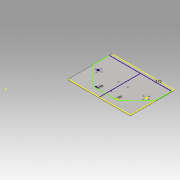
# Autodesk Inventor part: track side panel V1
Saved by Autodesk Inventor 2016 (Build 200138000, 138)
## iProperties
Created: 2015-10-10
Part Number: track side panel V1
Material: Generic
Document SubType Name: Modeling
Designer: Delta
Density: 1 g/cm^3
Appearance: Default
Author: Delta
Autodesk Inventor part; units mm, degrees
ref_plane "YZ Plane" through (0, 0, 0) normal (1, 0, 0) x (0, 1, 0)
ref_plane "XZ Plane" through (0, 0, 0) normal (0, 1, 0) x (-1, 0, 0)
ref_plane "XY Plane" through (0, 0, 0) normal (0, 0, 1) x (1, 0, 0)
sketch "Sketch1" plane through (0, 0, 0) normal (0, 1, 0) x (-1, 0, 0)
  line L0 (-77.6185, -139.5068) -> (-293.5185, -139.5068)
  line L1 (-293.5185, -139.5068) -> (-293.5185, -291.9068)
  line L2 (-293.5185, -291.9068) -> (-77.6185, -291.9068)
  line L3 (-77.6185, -291.9068) -> (-77.6185, -139.5068)
  point P0 (0, 0)
  dimension "d0" = 215.9
  dimension "d1" = 152.4
  constraints: 8 end point, 2 parallel, 1 horizontal, 1 perpendicular
  measures "d0" distance of L2.end L1.end
  measures "d1" distance of L1.end L0.end
extrude "Extrusion1" add sketch "Sketch1" along normal blind 3.175
sketch "Sketch2" plane through (0, 3.175, 0) normal (0, 1, 0) x (1, 0, 0)
  line L0 (77.6185, 291.9068) -> (77.6185, 139.5068) projected
  line L1 (77.6185, 139.5068) -> (293.5185, 139.5068) projected
  line L2 (293.5185, 139.5068) -> (293.5185, 291.9068) projected
  line L3 (293.5185, 291.9068) -> (77.6185, 291.9068) projected
  line L4 (185.5685, 291.9068) -> (185.5685, 139.5068)
  line L5 (104.9685, 218.5068) -> (221.9685, 218.5068) construction
  line L6 (156.9685, 165.5068) -> (156.9685, 258.7711) construction
  point P0 (0, 0)
  point P1 (269.9685, 218.5068)
  point P2 (221.9685, 165.5068)
  dimension "d4" = 144.35
  dimension "d5" = 26
  dimension "d7" = 79
  dimension "d19" = 27.35
  dimension "d20" = 79
  dimension "d21" = 26
  dimension "d22" = 79.35
  dimension "d23" = 192.35
  dimension "d180" = 65
  dimension "d201" = 36.4
  dimension "d202" = 28.6
  constraints: 6 end point, 2 midpoint, 1 horizontal, 1 vertical
  measures "d4" distance from line of L0 point (221.968, 165.507)
  measures "d5" distance from line of L1 point (221.968, 165.507)
  measures "d7" distance from line of L1 point (269.968, 218.507)
  measures "d19" distance from line of L0 L5.start
  measures "d20" distance from line of L1 L5.start
  measures "d21" distance from line of L1 L6.start
  measures "d22" distance from line of L0 L6.start
  measures "d23" distance from line of L0 point (269.968, 218.507)
  measures "d180" distance of L6.start point (221.968, 165.507)
  measures "d201" distance from line of L4 point (221.968, 165.507)
  measures "d202" distance from line of L4 L6.start
hole "Hole1" at (156.9685, 3.175, -165.5068) at (104.9685, 3.175, -218.5068) at (269.9685, 3.175, -218.5068) at (221.9685, 3.175, -165.5068) direction (0, -1, 0) diameter 6.35 end through all
sketch "Sketch3" plane through (0, 3.175, 0) normal (0, 1, 0) x (1, 0, 0)
  circle A0 centre (104.9685, 218.5068) radius 3.175 projected
  circle A1 centre (269.9685, 218.5068) radius 3.175 projected
  circle A2 centre (221.9685, 165.5068) radius 3.175 projected
  circle A3 centre (156.9685, 165.5068) radius 3.175 projected
  line L0 (293.5185, 139.5068) -> (293.5185, 291.9068) projected
  line L1 (77.6185, 139.5068) -> (293.5185, 139.5068) projected
  line L2 (104.9685, 218.5068) -> (156.9685, 165.5068) construction
  line L3 (78.5272, 236.3897) -> (154.4976, 158.9583)
  line L4 (185.5685, 291.9068) -> (185.5685, 139.5068) construction
  line L5 (185.5685, 158.0068) -> (156.7639, 158.0068)
  line L6 (80.7935, 282.3818) -> (185.5685, 282.3818)
  line L7 (77.6185, 279.2068) -> (77.6185, 238.6132)
  arc A4 (80.7935, 282.3818) -> (77.6185, 279.2068) centre (80.7935, 279.2068) ccw
  arc A5 (77.6185, 238.6132) -> (78.5272, 236.3897) centre (80.7935, 238.6132) ccw
  arc A6 (154.4976, 158.9583) -> (156.7639, 158.0068) centre (156.7639, 161.1818) ccw
  circle A7 centre (266.1685, 218.5068) radius 3.175
  circle A8 centre (214.1685, 165.5068) radius 3.175
  line L8 (266.1685, 218.5068) -> (214.1685, 165.5068) construction
  line L9 (292.6098, 236.3897) -> (216.6394, 158.9583)
  line L10 (185.5685, 158.0068) -> (214.3731, 158.0068)
  line L11 (290.3435, 282.3818) -> (185.5685, 282.3818)
  line L12 (293.5185, 279.2068) -> (293.5185, 238.6132)
  arc A9 (293.5185, 279.2068) -> (290.3435, 282.3818) centre (290.3435, 279.2068) ccw
  arc A10 (292.6098, 236.3897) -> (293.5185, 238.6132) centre (290.3435, 238.6132) ccw
  arc A11 (214.3731, 158.0068) -> (216.6394, 158.9583) centre (214.3731, 161.1818) ccw
  point P0 (0, 0)
  point P1 (77.6185, 237.3158)
  point P2 (77.6185, 282.3818)
  point P3 (293.5185, 237.3158)
  point P4 (293.5185, 282.3818)
  dimension "d192" = 6.35
  dimension "d193" = 7.5
  dimension "d197" = 3.175
  dimension "d198" = 3.175
  constraints: 22 end point, 14 symmetric about line, 12 point on circle, 10 point on line, 8 centre point, 6 tangent, 1 equal radius, 1 midpoint, 1 parallel, 1 perpendicular, 5 other
  measures "d192" distance between parallel lines of L2 L3
  measures "d193" distance from line of L5 point (156.968, 165.507)
  measures "d197" radius of A4
  measures "d198" radius of A5
extrude "Extrusion3" [suppressed]
sketch "Sketch7" plane through (0, 3.175, 0) normal (0, 1, 0) x (1, 0, 0)
  circle A0 centre (156.9685, 165.5068) radius 3.175 projected
  line L0 (155.9994, 158.0068) -> (221.9685, 158.0068) projected
  circle A1 centre (156.7936, 178.0024) radius 2.9972
  line L1 (153.7965, 177.9961) -> (153.7965, 165.3697)
  line L2 (159.7908, 178.0031) -> (160.1422, 165.5967)
  circle A2 centre (222.1463, 178.0024) radius 2.9972
  circle A3 centre (221.9685, 165.5068) radius 3.175 projected
  line L3 (219.1491, 178.0147) -> (219.1491, 164.0468)
  line L4 (225.1435, 178.0036) -> (225.1435, 165.5068)
  point P0 (0, 0)
  point P1 (218.7935, 165.5083)
  dimension "d76" = 5.9944
  dimension "d77" = 12.4968
  dimension "d78" = 5.9944
  dimension "d79" = 12.4968
  dimension "d88" = 6.35
  constraints: 9 point on circle, 8 end point, 3 vertical, 2 centre point, 1 tangent, 3 other
  measures "d76" diameter of A1
  measures "d77" distance of A0.centre A1.centre
  measures "d78" diameter of A2
  measures "d79" distance of A3.centre A2.centre
  measures "d88" diameter of A0
extrude "Extrusion4" cut sketch "Sketch7" against normal blind 25.4 contours A0 L1 A1 L2 | A1
sketch "Sketch8" plane through (0, 3.175, 0) normal (0, 1, 0) x (1, 0, 0)
  arc A0 (224.9685, 178.0036) -> (218.9741, 177.9913) centre (221.9713, 178.0036) ccw
  circle A1 centre (221.9685, 165.5068) radius 3
  line L0 (218.9741, 178.016) -> (218.9741, 165.3232)
  line L1 (224.9685, 178.0036) -> (224.9685, 165.5068)
  point P0 (0, 0)
  point P1 (218.9685, 165.5082)
  dimension "d82" = 5.9944
  dimension "d83" = 12.4968
  constraints: 6 point on circle, 4 end point, 2 centre point, 2 vertical, 1 point on line
  measures "d82" diameter of A0
  measures "d83" distance of A1.centre A0.centre
extrude "Extrusion5" cut sketch "Sketch8" against normal blind 25.4 contours L1 A1 L0 A0 | A1 L0 picked at (221.9464, 164.5591)
sketch "Sketch5" plane through (0, 3.175, 0) normal (0, 1, 0) x (1, 0, 0)
  circle A0 centre (104.9685, 218.5068) radius 3.175 projected
  circle A1 centre (104.9685, 218.5068) radius 22.225
  circle A2 centre (156.9685, 165.5068) radius 3.175 projected
  circle A3 centre (156.9685, 165.5068) radius 22.225
  circle A4 centre (221.9685, 165.5068) radius 3.175 projected
  circle A5 centre (221.9685, 165.5068) radius 22.225
  circle A6 centre (269.9685, 218.5068) radius 3.175 projected
  circle A7 centre (269.9685, 218.5068) radius 22.225
  line L0 (155.9994, 158.0068) -> (221.9685, 158.0068) projected
  arc A8 (224.9685, 178.0036) -> (218.9741, 178.016) centre (221.9713, 178.0036) ccw projected
  line L1 (287.1685, 282.4291) -> (83.9685, 282.4291) projected
  point P0 (0, 0)
  point P1 (205.7185, 218.5096)
  point P2 (189.4685, 178.0036)
  point P3 (173.2185, 218.5096)
  dimension "d45" = 44.45
  dimension "d47" = 44.45
  dimension "d48" = 44.45
  dimension "d49" = 44.45
  dimension "d50" = 60.5028
  dimension "d52" = 65
  dimension "d53" = 16.25
  dimension "d54" = 16.25
  dimension "d55" = 60.5028
  dimension "d58" = 52
  dimension "d62" = 32.5
  dimension "d125" = 0
  dimension "d181" = 32.5
  dimension "d186" = 63.9194
  constraints: 4 centre point, 4 coincident
  measures "d45" diameter of A1
  measures "d47" diameter of A3
  measures "d48" diameter of A5
  measures "d49" diameter of A7
  measures "d50" distance from line of L0 point (173.218, 218.51)
  measures "d52" distance of A5.centre A3.centre
  measures "d53" horizontal distance of point (173.218, 218.51) A3.centre
  measures "d54" horizontal distance of A5.centre point (205.718, 218.51)
  measures "d55" distance from line of L0 point (205.718, 218.51)
  measures "d58" horizontal distance of A3.centre A1.centre
  measures "d62" horizontal distance of A3.centre point (189.468, 178.004)
  measures "d125" vertical distance of A8.centre point (189.468, 178.004)
  measures "d181" distance of point (205.718, 218.51) point (173.218, 218.51)
  measures "d186" distance from line of L1 point (173.218, 218.51)
hole "Hole2" at (205.7185, 3.175, -218.5096) at (189.4685, 3.175, -178.0036) at (173.2185, 3.175, -218.5096) direction (0, -1, 0) diameter 3 end through all
sketch "Sketch11" plane through (0, 3.175, 0) normal (0, 1, 0) x (1, 0, 0)
  circle A0 centre (104.9685, 218.5068) radius 3.175 projected
  circle A1 centre (104.9685, 218.5068) radius 9.7333
  line L0 (95.2722, 217.6585) -> (104.1202, 228.2031) construction
  line L1 (79.8868, 220.4869) -> (153.2717, 158.9097) construction
  circle A2 centre (269.9685, 218.5068) radius 9.7333
  line L2 (269.0987, 208.8124) -> (279.6629, 217.6371) construction
  line L3 (227.8466, 160.8487) -> (291.2394, 213.8031) construction
  point P0 (105.8168, 208.8105)
  point P1 (114.6648, 219.3552)
  point P2 (270.8383, 228.2012)
  point P3 (260.2741, 219.3766)
  dimension "d174" = 19.4667
  dimension "d175" = 19.4667
  dimension "d161" = 360
  dimension "d178" = 360
  constraints: 4 end point, 2 coincident, 1 parallel, 1 perpendicular, 16 other
hole "Hole4" at (95.2722, 3.175, -217.6585) at (105.8168, 3.175, -208.8105) at (114.6648, 3.175, -219.3552) at (104.1202, 3.175, -228.2031) at (260.2741, 3.175, -219.3766) at (270.8383, 3.175, -228.2012) at (279.6629, 3.175, -217.6371) at (269.0987, 3.175, -208.8124) direction (0, -1, 0) diameter 2.7178 end through all
sketch "Sketch15" plane through (0, 3.175, 0) normal (0, 1, 0) x (1, 0, 0)
  circle A0 centre (269.9685, 218.5068) radius 3.175 projected
  arc A1 (218.9741, 166.5625) -> (224.9685, 166.5464) centre (221.9685, 165.5068) ccw projected
  line L0 (226.6751, 161.2442) -> (185.5685, 161.2442)
  line L1 (293.5185, 291.9068) -> (77.6185, 291.9068) projected
  line L2 (185.5685, 282.3818) -> (185.5685, 139.5068)
  line L3 (77.6185, 139.5068) -> (293.5185, 139.5068) projected
  line L4 (226.6751, 161.2442) -> (293.5185, 225.5385)
  line L5 (293.5185, 282.3818) -> (185.5685, 282.3818)
  line L6 (293.5185, 282.3818) -> (293.5185, 225.5385)
  line L7 (293.5185, 139.5068) -> (293.5185, 291.9068) projected
  circle A2 centre (101.1685, 218.5068) radius 3.175
  arc A3 (146.1685, 166.5464) -> (152.1629, 166.5625) centre (149.1685, 165.5068) ccw
  line L8 (144.4618, 161.2442) -> (185.5685, 161.2442)
  line L9 (144.4618, 161.2442) -> (77.6185, 225.5385)
  line L10 (77.6185, 282.3818) -> (185.5685, 282.3818)
  line L11 (77.6185, 282.3818) -> (77.6185, 225.5385)
  point P0 (0, 0)
  dimension "d200" = 9.525
  constraints: 18 end point, 7 symmetric about line, 2 centre point, 2 point on circle, 1 collinear, 1 horizontal, 1 midpoint, 1 perpendicular, 1 point on line, 1 vertical, 2 other
  measures "d200" distance between parallel lines of L1 L5
equation "\"d78\" = d76"
equation "\"d79\" = d77"
equation "\"d82\" = d84"
equation "\"d83\" = d85"
equation "\"d47\" = d45"
equation "\"d48\" = d45"
equation "\"d49\" = d48"
equation "\"d53\" = 0.25 * d52"
equation "\"d54\" = d53"
equation "\"d55\" = d50"
equation "\"d62\" = 0.5 * d52"
equation "\"d84\" = 5.9944"
equation "\"d85\" = 12.4968"
body "Solid1"
